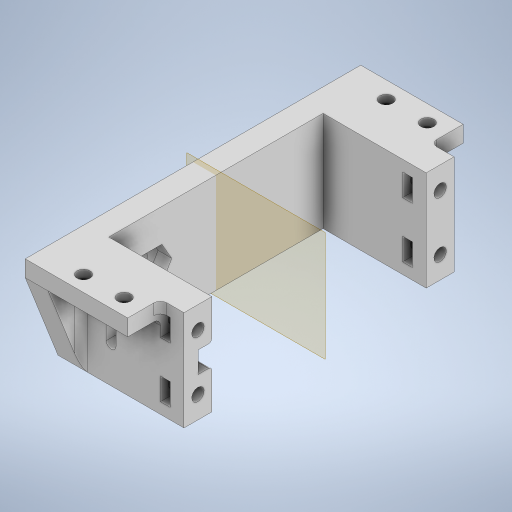
# Autodesk Inventor part: wheelie
Saved by Autodesk Inventor 2024 (Build 280153020, 153B)
## iProperties
Created: 2024-02-29
Part Number: wheelie
Material: Generic
Document SubType Name: Modeling
Designer: 5802269
Density: 1 g/cm^3
Appearance: Default
Author: 5802269
Autodesk Inventor part; units mm, degrees
ref_plane "YZ Plane" through (0, 0, 0) normal (1, 0, 0) x (0, 1, 0)
ref_plane "XZ Plane" through (0, 0, 0) normal (0, 1, 0) x (-1, 0, 0)
ref_plane "XY Plane" through (0, 0, 0) normal (0, 0, 1) x (1, 0, 0)
sketch "Sketch2" plane through (0, 0, 0) normal (1, 0, 0) x (0, 1, 0)
  line L0 (-15.25, -41.25) -> (15.25, -41.25)
  line L1 (15.25, -41.25) -> (15.25, 41.25)
  line L2 (15.25, 41.25) -> (-15.25, 41.25)
  line L3 (-15.25, 41.25) -> (-15.25, -41.25)
  line L4 (-15.25, -41.25) -> (15.25, 41.25) construction
  line L5 (15.25, -41.25) -> (-15.25, 41.25) construction
  line L6 (-15.25, 32.75) -> (15.25, 32.75)
  line L7 (15.25, 32.75) -> (15.25, -32.75)
  line L8 (15.25, -32.75) -> (-15.25, -32.75)
  line L9 (-15.25, -32.75) -> (-15.25, 32.75)
  line L10 (-15.25, 32.75) -> (15.25, -32.75) construction
  line L11 (15.25, 32.75) -> (-15.25, -32.75) construction
  line L12 (0, 41.25) -> (0, 37) construction
  line L13 (0, 37) -> (8.5, 37) construction
  line L14 (8.5, 37) -> (0, 37) construction
  line L15 (0, 37) -> (-8.5, 37) construction
  line L16 (15.25, 0) -> (-15.25, 0) construction
  circle A0 centre (8.5, 37) radius 1.9
  circle A1 centre (8.5, -37) radius 1.9
  line L17 (0, -41.25) -> (0, 41.25) construction
  circle A2 centre (-8.5, 37) radius 1.9
  circle A3 centre (-8.5, -37) radius 1.9
  point P0 (0, 0)
  dimension "d0" = 30.5
  dimension "d1" = 82.5
  dimension "d2" = 30.5
  dimension "d3" = 65.5
  dimension "d4" = 4.25
  dimension "d6" = 8.5
  dimension "d7" = 8.5
  dimension "d8" = 8.5
  dimension "d14" = 3.8
  constraints: 36 end point, 8 midpoint, 5 equal length, 4 centre point, 3 horizontal, 3 perpendicular, 3 symmetric about line, 1 coincident, 1 point on line, 1 vertical, 3 other
  measures "d0" distance of L2.end L1.end
  measures "d1" distance of L1.end L0.end
  measures "d2" distance of L7.end L8.end
  measures "d3" distance of L6.end L7.end
  measures "d4" distance of L12.start L12.end
  measures "d6" distance of L12.end L13.end
  measures "d7" distance of L13.end L12.end
  measures "d8" distance of L12.end L15.end
  measures "d14" diameter of A0
extrude "Extrusion2" add sketch "Sketch2" along normal blind 31.5 contours L3 L8 L1 L0 | L3 L2 L1 L6
sketch "Sketch4" plane through (0, 0, 0) normal (-1, 0, 0) x (0, 0, 1)
  circle A0 centre (-37, 8.5) radius 1.9 projected
  circle A1 centre (-37, 8.5) radius 1.9
  circle A2 centre (-37, -8.5) radius 1.9 projected
  circle A3 centre (-37, -8.5) radius 1.9
  circle A4 centre (37, 8.5) radius 1.9 projected
  circle A5 centre (37, 8.5) radius 1.9
  circle A6 centre (37, -8.5) radius 1.9 projected
  circle A7 centre (37, -8.5) radius 1.9
  point P0 (0, 0)
  constraints: 4 centre point, 4 coincident
extrude "Extrusion3" add sketch "Sketch4" against normal blind 23.5
sketch "Sketch5" plane through (0, 0, 0) normal (-1, 0, 0) x (0, 0, 1)
  line L0 (-41.25, -15.25) -> (-41.25, 15.25) projected
  line L1 (41.25, 15.25) -> (41.25, -15.25) projected
  line L2 (-41.25, 15.25) -> (41.25, 15.25)
  line L3 (41.25, 15.25) -> (41.25, -15.25)
  line L4 (41.25, -15.25) -> (-41.25, -15.25)
  line L5 (-41.25, -15.25) -> (-41.25, 15.25)
  point P0 (0, 0)
  constraints: 8 end point, 2 parallel, 1 horizontal, 1 perpendicular
extrude "Extrusion4" add sketch "Sketch5" along normal blind 7
sketch "Sketch8" plane through (0, 0, 0) normal (1, 0, 0) x (0, 0, -1)
  line L0 (-32.75, -15.25) -> (-32.75, 15.25) construction
  line L1 (-32.75, 0) -> (-19.55, 0) construction
  line L2 (-19.55, 0) -> (-19.55, -5.25) construction
  line L3 (-22.5811, -5.25) -> (-25.6122, 0)
  line L4 (-25.6122, 0) -> (-22.5811, 5.25)
  line L5 (-22.5811, 5.25) -> (-16.5189, 5.25)
  line L6 (-16.5189, 5.25) -> (-13.4878, 0)
  line L7 (-13.4878, 0) -> (-16.5189, -5.25)
  line L8 (-16.5189, -5.25) -> (-22.5811, -5.25)
  point P0 (0, 0)
  dimension "d25" = 13.2
  dimension "d26" = 5.25
  constraints: 16 end point, 2 midpoint, 1 coincident, 1 horizontal, 1 vertical, 13 other
  measures "d25" distance of L1.start L1.end
  measures "d26" distance of L1.end L2.end
extrude "Extrusion6" cut sketch "Sketch8" against normal blind 4.2
sketch "Sketch9" plane through (-4.2, 0, 0) normal (1, 0, 0) x (0, 0, -1)
  circle A0 centre (-19.55, 0) radius 2.875
  point P0 (0, 0)
  dimension "d29" = 5.75
  constraints: 1 centre point
  measures "d29" diameter of A0
extrude "Extrusion7" cut sketch "Sketch9" against normal through all
sketch "Sketch10" plane through (31.5, -15.25, 32.75) normal (0, 0, -1) x (-1, 0, 0)
  line L0 (0, 0) -> (0, 30.5) projected
  line L1 (31.5, 30.5) -> (0, 30.5) projected
  line L2 (23.75, 19.25) -> (23.75, 11.25)
  line L3 (20.75, 11.25) -> (20.75, 19.25)
  arc A0 (23.75, 19.25) -> (20.75, 19.25) centre (22.25, 19.25) ccw
  arc A1 (20.75, 11.25) -> (23.75, 11.25) centre (22.25, 11.25) ccw
  point P0 (31.5, 15.25)
  constraints: 4 end point, 4 point on circle, 2 centre point
extrude "Extrusion9" cut sketch "Sketch10" against normal through all
sketch "Sketch12" plane through (31.5, 0, 0) normal (1, 0, 0) x (0, 0, -1)
  line L0 (-32.75, -4) -> (-32.75, 4) projected
  line L1 (-32.75, 0) -> (-32.75, -3.25)
  line L2 (-32.75, -4) -> (-41.25, -4) projected
  line L3 (-32.75, -3.25) -> (-36.95, -3.25)
  line L4 (-36.95, -3.25) -> (-36.95, 0)
  line L5 (-36.95, 0) -> (-36.95, 3.25)
  line L6 (-36.95, 3.25) -> (-32.75, 3.25)
  line L7 (-32.75, 3.25) -> (-36.95, 3.25)
  line L8 (-36.95, 3.25) -> (-36.95, -3.25)
  line L9 (-36.95, -3.25) -> (-32.75, -3.25)
  line L10 (-32.75, -3.25) -> (-32.75, 3.25)
  point P0 (0, 0)
  dimension "d44" = 3.25
  dimension "d46" = 4.2
  dimension "d47" = 3.25
  dimension "d48" = 3.25
  dimension "d49" = 4.2
  constraints: 18 end point, 3 point on line, 2 horizontal, 2 parallel, 2 perpendicular, 1 midpoint
  measures "d44" distance of L1.start L1.end
  measures "d46" distance of L1.end L3.end
  measures "d47" distance of L3.end L4.end
  measures "d48" distance of L4.end L5.end
  measures "d49" distance of L5.end L6.end
extrude "Extrusion10" cut sketch "Sketch12" against normal up to surface (23.75 mm away)
fillet "Fillet1" radius 1 4 edges at (21.125, -3.25, 32.75) (21.125, 3.25, 32.75) (10.75, 3.25, 34.85) (10.75, -3.25, 34.85)
sketch "Sketch13" plane through (0, -15.25, 32.75) normal (0, 0, -1) x (-1, 0, 0)
  line L0 (-10.729, 19.5) -> (-31.5, 19.5) projected
  line L1 (0, 15.25) -> (-36.7981, 15.25) construction
  line L2 (-31.5, 19.5) -> (-31.5, 30.5) construction
  line L3 (7, 30.5) -> (-31.5, 30.5) construction
  line L4 (-31.5, 4.85) -> (-31.5, 8.65) construction
  line L5 (-31.5, 4.85) -> (-23.5, 4.85) construction
  line L6 (-31.5, 6.75) -> (-27.3, 6.75) construction
  line L7 (-23.5, 4.85) -> (-23.5, 8.65) construction
  line L8 (-27.3, 6.75) -> (-27.3, 10.15)
  line L9 (-27.3, 10.15) -> (-24.3, 10.15)
  line L10 (-24.3, 10.15) -> (-24.3, 3.35)
  line L11 (-24.3, 3.35) -> (-27.3, 3.35)
  line L12 (-27.3, 3.35) -> (-27.3, 6.75)
  line L13 (-27.3, 23.75) -> (-27.3, 20.35)
  line L14 (-27.3, 20.35) -> (-24.3, 20.35)
  line L15 (-24.3, 20.35) -> (-24.3, 27.15)
  line L16 (-24.3, 27.15) -> (-27.3, 27.15)
  line L17 (-27.3, 27.15) -> (-27.3, 23.75)
  dimension "d61" = 4.2
  dimension "d62" = 3.4
  dimension "d63" = 3
  dimension "d64" = 6.8
  dimension "d65" = 3
  dimension "d66" = 3.4
  constraints: 24 end point, 5 symmetric about line, 4 perpendicular, 2 point on line, 1 horizontal, 1 midpoint
  measures "d61" distance of L6.start L6.end
  measures "d62" distance of L6.end L8.end
  measures "d63" distance of L8.end L9.end
  measures "d64" distance of L9.end L10.end
  measures "d65" distance of L10.end L11.end
  measures "d66" distance of L11.end L6.end
extrude "Extrusion12" cut sketch "Sketch13" along normal through all both and the other way through all
sketch "Sketch16" plane through (31.5, -15.25, -41.25) normal (0, 0, -1) x (-1, 0, 0)
  line L0 (7.2, 27.15) -> (7.2, 20.35) construction
  line L1 (7.2, 27.15) -> (7.2, 30.5) construction
  line L2 (31.5, 30.5) -> (0, 30.5) construction
  line L3 (7.2, 30.5) -> (15.025, 30.5) construction
  line L4 (7.2, 30.5) -> (15.2, 30.5)
  line L5 (7.2, 21.7029) -> (7.2, 30.5)
  line L6 (38.5, 30.5) -> (38.5, 0) projected
  line L7 (7.2, 30.5) -> (38.5, 30.5)
  line L8 (38.5, 30.5) -> (38.5, 25.5)
  line L9 (38.5, 25.5) -> (7.2, 25.5)
  line L10 (7.2, 25.5) -> (7.2, 30.5)
  point P0 (31.5, 15.25)
  dimension "d76" = 5
  constraints: 16 end point, 3 point on line, 2 horizontal, 2 parallel, 1 perpendicular, 1 vertical
  measures "d76" distance of L7.end L8.end
extrude "Extrusion13" add sketch "Sketch16" along normal blind 10
ref_plane "Work Plane1" through (31.5, -15.25, 0) normal (0, 0, 1) x (1, 0, 0)
mirror "Mirror1" about plane through (31.5, -15.25, 0) normal (0, 0, 1) of "Extrusion13"
sketch "Sketch18" plane through (-7, 0, 0) normal (-1, 0, 0) x (0, 0, 1)
  line L0 (-41.25, 10.25) -> (-51.25, 10.25) projected
  line L1 (-41.25, -15.25) -> (-41.25, 15.25) projected
  line L2 (-51.25, 10.25) -> (-41.25, -15.25)
  line L3 (41.25, 10.25) -> (51.25, 10.25) projected
  line L4 (41.25, -15.25) -> (41.25, 10.25) projected
  line L5 (51.25, 10.25) -> (41.25, -15.25)
  point P0 (0, 0)
  point P1 (-43.25, 10.25)
  constraints: 4 end point
extrude "Extrusion14" add sketch "Sketch18" against normal blind 7
fillet "Fillet3" radius 2 6 edges at (12.15, 10.25, -41.25) (24.3, 13.575, -41.25) (0, -2.5, -41.25) (0, -2.5, 41.25) (12.15, 10.25, 41.25) (24.3, 13.575, 41.25)
sketch "Sketch19" plane through (0, 10.25, -51.25) normal (0, -1, 0) x (1, 0, 0)
  point P0 (0, 51.25)
  point P1 (18.4468, 5.1027)
  point P2 (6.0056, 5.2269)
  point P3 (18.3492, 97.6405)
  point P4 (6.0592, 97.7607)
hole "Hole1" at (18.4468, 10.25, -46.1473) at (6.0056, 10.25, -46.0231) at (18.3492, 10.25, 46.3905) at (6.0592, 10.25, 46.5107) direction (0, 1, 0) diameter 4 end through all start extended yes countersink diameter 9.2 countersink angle 90
body "Solid2"
